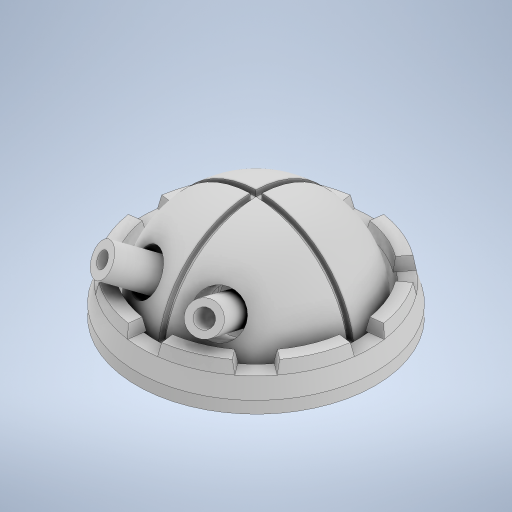
# Autodesk Inventor part: 屋頂-2
Saved by Autodesk Inventor 2024 (Build 280153000, 153)
## iProperties
Created: 2024-05-18
Part Number: 屋頂-2
Material: 一般
Document SubType Name: Modeling
Designer: User
Density: 1 g/cm^3
Appearance: 預設
Author: User
Autodesk Inventor part; units mm, degrees
ref_plane "YZ Plane" through (0, 0, 0) normal (1, 0, 0) x (0, 1, 0)
sketch "草圖1" plane through (0, 0, 0) normal (0, 1, 0) x (-1, 0, 0)
  circle A0 centre (0, 0) radius 16
  circle A1 centre (0, 0) radius 20
  line L0 (0, 16) -> (0, -16)
  dimension "d0" = 32
  dimension "d1" = 40
  constraints: 2 centre point, 2 coincident, 2 end point, 2 point on circle, 1 vertical
  measures "d0" diameter of A0
  measures "d1" diameter of A1
sketch "草圖1 outline for 迴轉1" plane through (0, 0, 0) normal (0, 1, 0) x (-1, 0, 0)
  line L0 (0, -16) -> (0, 16)
  arc A0 (0, 16) -> (0, -16) centre (0, 0) ccw
revolve "迴轉1" add sketch "草圖1 outline for 迴轉1" angle 180 about axis through (0, 0, 16) along (0, 0, 1)
sketch "草圖3" plane through (0, 0, 0) normal (1, 0, 0) x (0, 1, 0)
  line L0 (2, -15.874508) -> (2, 15.874508)
  arc A0 (2, -15.874508) -> (2, 15.874508) centre (0, 0) ccw
  arc A1 (1.774523, -14.894666) -> (1.774523, 14.894666) centre (0, 0) ccw
  line L1 (2, 15.874508) -> (2, -15.874508)
  point P0 (0, 0)
  point P1 (2, 14.866069)
  point P2 (2, -14.866069)
  dimension "d9" = 1
  constraints: 4 point on circle, 2 centre point, 2 end point, 1 concentric, 1 vertical
  measures "d9" radial gap between concentric circles of A0 A1
sketch "草圖3 outline for 擠出2" plane through (0, 0, 0) normal (1, 0, 0) x (0, 1, 0)
  arc A0 (2, -15.874508) -> (2, 15.874508) centre (0, 0) ccw
  line L0 (2, -14.866069) -> (2, -15.874508)
  arc A1 (2, 14.866069) -> (2, -14.866069) centre (0, 0) cw
  line L1 (2, 15.874508) -> (2, 14.866069)
extrude "擠出2" cut sketch "草圖3 outline for 擠出2" along normal mid plane 1
sketch "草圖4" plane through (0, 0, 0) normal (0, 0, 1) x (1, 0, 0)
  line L0 (15.874508, 2) -> (0.5, 2)
  line L1 (-0.5, 2) -> (-15.874508, 2)
  arc A0 (15.874508, 2) -> (-15.874508, 2) centre (0, 0) ccw
  arc A1 (16, 0) -> (-16, 0) centre (0, 0) ccw
  line L2 (20, 2) -> (-20, 2)
  arc A2 (14.866069, 2) -> (-14.866069, 2) centre (0, 0) ccw
  line L3 (-15.874508, 2) -> (16, 2)
  point P0 (-14.866069, 2)
  dimension "d13" = 1
  constraints: 4 point on circle, 2 centre point, 2 concentric, 2 end point, 1 horizontal, 4 other
  measures "d13" radial gap between concentric circles of A0 A2
sketch "草圖4 outline for 擠出3" plane through (0, 0, 0) normal (0, 0, 1) x (1, 0, 0)
  arc A0 (-14.866069, 2) -> (14.866069, 2) centre (0, 0) cw
  line L0 (-15.874508, 2) -> (-14.866069, 2)
  arc A1 (15.874508, 2) -> (-15.874508, 2) centre (0, 0) ccw
  line L1 (14.866069, 2) -> (15.874508, 2)
extrude "擠出3" cut sketch "草圖4 outline for 擠出3" along normal mid plane 1
sketch "草圖6" plane through (0, 0, 0) normal (0, -1, 0) x (1, 0, 0)
  circle A0 centre (0, 0) radius 16
  circle A1 centre (0, 0) radius 20
  dimension "d22" = 32
  dimension "d23" = 40
  constraints: 2 centre point, 2 coincident
  measures "d22" diameter of A0
  measures "d23" diameter of A1
sketch "草圖6 outline for 擠出5" plane through (0, 0, 0) normal (0, -1, 0) x (1, 0, 0)
  circle A0 centre (0, 0) radius 16
extrude "擠出5" add sketch "草圖6 outline for 擠出5" along normal blind 2
sketch "草圖6 outline for 擠出6" plane through (0, 0, 0) normal (0, -1, 0) x (1, 0, 0)
  circle A0 centre (0, 0) radius 20
  circle A1 centre (0, 0) radius 16
extrude "擠出6" add sketch "草圖6 outline for 擠出6" along normal blind 2 and the other way blind 3 draft -15
sketch "草圖7" plane through (0, 3, 0) normal (0, 1, 0) x (1, 0, 0)
  line L0 (0, 0) -> (2.505601, 19.031927)
  circle A0 centre (0, 0) radius 19.196152
  line L1 (0, 0) -> (11.685877, 15.229332)
  line L2 (0, 0) -> (15.229332, 11.685877)
  line L3 (0, 0) -> (19.031927, 2.505601)
  line L4 (0.5, 0.5) -> (0.5, 15.866632)
  line L5 (0, 0) -> (-19.031927, 2.505601)
  line L6 (0, 0) -> (-15.229332, 11.685877)
  line L7 (0, 0) -> (-11.685877, 15.229332)
  line L8 (0, 0) -> (-2.505601, 19.031927)
  line L9 (0, 0) -> (-2.505601, -19.031927)
  line L10 (0, 0) -> (-11.685877, -15.229332)
  line L11 (0, 0) -> (-15.229332, -11.685877)
  line L12 (0, 0) -> (-19.031927, -2.505601)
  line L13 (0, 0) -> (19.031927, -2.505601)
  line L14 (0, 0) -> (15.229332, -11.685877)
  line L15 (0, 0) -> (11.685877, -15.229332)
  line L16 (0, 0) -> (2.505601, -19.031927)
  circle A1 centre (0, 0) radius 16.401924
  circle A2 centre (0, 0) radius 19.196152
  point P0 (13.012521, 9.984859)
  point P1 (16.261603, 2.140881)
  point P2 (16.261603, -2.140881)
  point P3 (13.012521, -9.984859)
  point P4 (15.229332, -11.685877)
  point P5 (9.984859, -13.012521)
  point P6 (2.140881, -16.261603)
  point P7 (2.505601, -19.031927)
  point P8 (11.685877, -15.229332)
  point P9 (-2.140881, -16.261603)
  point P10 (-9.984859, -13.012521)
  point P11 (-11.685877, -15.229332)
  point P12 (-13.012521, -9.984859)
  point P13 (-16.261603, -2.140881)
  point P14 (-19.031927, -2.505601)
  point P15 (-15.229332, -11.685877)
  point P16 (-16.261603, 2.140881)
  point P17 (-13.012521, 9.984859)
  point P18 (-19.031927, 2.505601)
  point P19 (-9.984859, 13.012521)
  point P20 (-2.140881, 16.261603)
  point P21 (-2.505601, 19.031927)
  point P22 (-11.685877, 15.229332)
  point P23 (2.140881, 16.261603)
  point P24 (9.984859, 13.012521)
  dimension "d30" = 30
  dimension "d31" = 30
  dimension "d32" = 15
  dimension "d37" = 360
  constraints: 32 end point, 4 coincident, 4 point on circle, 2 centre point, 1 concentric, 39 other
  measures "d30" angle of L1 L0
  measures "d31" angle of L3 L2
  measures "d32" angle of L2 L1
sketch "草圖7 outline for 擠出7" plane through (0, 3, 0) normal (0, 1, 0) x (1, 0, 0)
  arc A0 (13.012521, 9.984859) -> (16.261603, 2.140881) centre (0, 0) cw
  line L0 (15.229332, 11.685877) -> (13.012521, 9.984859)
  arc A1 (19.031927, 2.505601) -> (15.229332, 11.685877) centre (0, 0) ccw
  line L1 (16.261603, 2.140881) -> (19.031927, 2.505601)
  arc A2 (16.261603, -2.140881) -> (13.012521, -9.984859) centre (0, 0) cw
  line L2 (19.031927, -2.505601) -> (16.261603, -2.140881)
  arc A3 (15.229332, -11.685877) -> (19.031927, -2.505601) centre (0, 0) ccw
  line L3 (13.012521, -9.984859) -> (15.229332, -11.685877)
  arc A4 (9.984859, -13.012521) -> (2.140881, -16.261603) centre (0, 0) cw
  line L4 (11.685877, -15.229332) -> (9.984859, -13.012521)
  arc A5 (2.505601, -19.031927) -> (11.685877, -15.229332) centre (0, 0) ccw
  line L5 (2.140881, -16.261603) -> (2.505601, -19.031927)
  arc A6 (-2.140881, -16.261603) -> (-9.984859, -13.012521) centre (0, 0) cw
  line L6 (-2.505601, -19.031927) -> (-2.140881, -16.261603)
  arc A7 (-11.685877, -15.229332) -> (-2.505601, -19.031927) centre (0, 0) ccw
  line L7 (-9.984859, -13.012521) -> (-11.685877, -15.229332)
  arc A8 (-13.012521, -9.984859) -> (-16.261603, -2.140881) centre (0, 0) cw
  line L8 (-15.229332, -11.685877) -> (-13.012521, -9.984859)
  arc A9 (-19.031927, -2.505601) -> (-15.229332, -11.685877) centre (0, 0) ccw
  line L9 (-16.261603, -2.140881) -> (-19.031927, -2.505601)
  arc A10 (-16.261603, 2.140881) -> (-13.012521, 9.984859) centre (0, 0) cw
  line L10 (-19.031927, 2.505601) -> (-16.261603, 2.140881)
  arc A11 (-15.229332, 11.685877) -> (-19.031927, 2.505601) centre (0, 0) ccw
  line L11 (-13.012521, 9.984859) -> (-15.229332, 11.685877)
  arc A12 (-9.984859, 13.012521) -> (-2.140881, 16.261603) centre (0, 0) cw
  line L12 (-11.685877, 15.229332) -> (-9.984859, 13.012521)
  arc A13 (-2.505601, 19.031927) -> (-11.685877, 15.229332) centre (0, 0) ccw
  line L13 (-2.140881, 16.261603) -> (-2.505601, 19.031927)
  arc A14 (2.140881, 16.261603) -> (9.984859, 13.012521) centre (0, 0) cw
  line L14 (2.505601, 19.031927) -> (2.140881, 16.261603)
  arc A15 (11.685877, 15.229332) -> (2.505601, 19.031927) centre (0, 0) ccw
  line L15 (9.984859, 13.012521) -> (11.685877, 15.229332)
extrude "擠出7" add sketch "草圖7 outline for 擠出7" along normal blind 2 draft -10
ref_plane "工作平面7" through (0, 0, 0) normal (0.3870815, -0.4851124, -0.7841134) x (0.7816608, 0.6237038, 0)
ref_plane "工作平面8" through (0, 0, 0) normal (0.3887941, 0.4847331, 0.7835004) x (-0.7800772, 0.6256833, 0)
sketch "草圖14" plane through (0, 0, 0) normal (0.3870815, -0.4851124, -0.7841134) x (0.7816608, 0.6237038, 0)
  line L0 (-3.118519, 3.064554) -> (0, 0)
  circle A0 centre (0, 0) radius 2.6
  dimension "d70" = 5.2
  constraints: 1 centre point, 1 coincident
  measures "d70" diameter of A0
sketch "草圖14 outline for 擠出15" plane through (0, 0, 0) normal (0.3870815, -0.4851124, -0.7841134) x (0.7816608, 0.6237038, 0)
  circle A0 centre (0, 0) radius 2.6
extrude "擠出15" add sketch "草圖14 outline for 擠出15" against normal blind 22
sketch "草圖15" plane through (-8.515794, 10.672472, 17.250495) normal (-0.3870815, 0.4851124, 0.7841134) x (0.8966914, 0, 0.4426562)
  circle A0 centre (0, 0) radius 3.5
  circle A1 centre (0, 0) radius 1.25
  circle A2 centre (0, 0) radius 2.6
  point P0 (0, 0)
  dimension "d73" = 7
  dimension "d74" = 2.5
  dimension "d77" = 5.2
  constraints: 3 centre point, 3 coincident
  measures "d73" diameter of A0
  measures "d74" diameter of A1
  measures "d77" diameter of A2
sketch "草圖15 outline for 擠出16" plane through (-8.515794, 10.672472, 17.250495) normal (-0.3870815, 0.4851124, 0.7841134) x (0.8966914, 0, 0.4426562)
  circle A0 centre (0, 0) radius 1.25
extrude "擠出16" cut sketch "草圖15 outline for 擠出16" against normal blind 10
sketch "草圖15 outline for 擠出17" plane through (-8.515794, 10.672472, 17.250495) normal (-0.3870815, 0.4851124, 0.7841134) x (0.8966914, 0, 0.4426562)
  circle A0 centre (0, 0) radius 3.5
  circle A1 centre (0, 0) radius 2.6
extrude "擠出17" cut sketch "草圖15 outline for 擠出17" against normal blind 15
sketch "草圖16" plane through (0, 0, 0) normal (0.3887941, 0.4847331, 0.7835004) x (-0.7800772, 0.6256833, 0)
  circle A0 centre (0, 0) radius 2.5
  dimension "d80" = 5
  constraints: 1 centre point, 1 coincident
  measures "d80" diameter of A0
sketch "草圖16 outline for 擠出18" plane through (0, 0, 0) normal (0.3887941, 0.4847331, 0.7835004) x (-0.7800772, 0.6256833, 0)
  circle A0 centre (0, 0) radius 2.5
extrude "擠出18" add sketch "草圖16 outline for 擠出18" along normal blind 22
sketch "草圖17" plane through (8.55347, 10.664129, 17.23701) normal (0.3887941, 0.4847331, 0.7835004) x (0.895775, 0, -0.4445078)
  circle A0 centre (0, 0) radius 1.4
  circle A1 centre (0, 0) radius 2.5
  circle A2 centre (0, 0) radius 3.5
  point P0 (0, 0)
  dimension "d83" = 2.8
  dimension "d84" = 5
  dimension "d85" = 7
  constraints: 3 centre point, 3 coincident
  measures "d83" diameter of A0
  measures "d84" diameter of A1
  measures "d85" diameter of A2
sketch "草圖17 outline for 擠出19" plane through (8.55347, 10.664129, 17.23701) normal (0.3887941, 0.4847331, 0.7835004) x (0.895775, 0, -0.4445078)
  circle A0 centre (0, 0) radius 1.4
extrude "擠出19" cut sketch "草圖17 outline for 擠出19" against normal blind 10
sketch "草圖17 outline for 擠出20" plane through (8.55347, 10.664129, 17.23701) normal (0.3887941, 0.4847331, 0.7835004) x (0.895775, 0, -0.4445078)
  circle A0 centre (0, 0) radius 3.5
  circle A1 centre (0, 0) radius 2.5
extrude "擠出20" cut sketch "草圖17 outline for 擠出20" against normal blind 15
